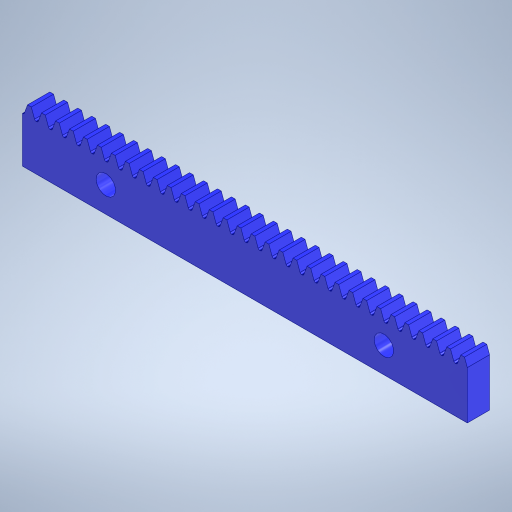
# Autodesk Inventor part: LRGEAM0.8KA-80-K2-B50
Saved by Autodesk Inventor 2024 (Build 280153000, 153)
## iProperties
Category: PARTsolutions
Company: MISUMI
Created: 2025-06-07
Part Number: LRGEAM0.8KA-80-K2-B50
Material: ナイロン 6
Catalog Web Link: www.cadenas.de
Description: LRGEA, LRGEAS,LRGEAB,LRGEAM,LRGEAP-Rack Gears L Dimension Configurable (One End Machined) - Pressure Angle 20 - Hole Qty. Configurable
Vendor: MISUMI
Document SubType Name: Modeling
Designer: psAdmin
Manufacturer: MISUMI
Mass: 3.19789 g
Surface Area: 25.3066 cm^2
Volume: 2.85525 cm^3
Density: 1.12 g/cm^3
Appearance: 青 - 壁塗料 - 光沢
PSOL_IDENT_0: {$CADENAS_DATA/23d-libs/misumi/metric/54_spur_gears/lrgea.prj},252 {VTYP=3D},{NB=LRGEAM0.8KA-80-K2-B
PSOL_IDENT_1: 50},{LINA=LRGEAM0.8KA-80-K2-B50},{NN=LRGEA, LRGEAS,LRGEAB,LRGEAM,LRGEAP},{DATE=29.05.2023 09:31:19},
PSOL_IDENT_2: {GEOMDATE=04.08.2020 02:33:51},{VERSION=},{LINEID=80},{WBVAR=MAT,L,HM,K,B,ALT1,ALT2,MS,ALT3,TPC},{WB
PSOL_IDENT_3: NUMERIC=L,K,B,MS}  {NB=LRGEAM0.8KA-80-K2-B50},{LINA=LRGEAM0.8KA-80-K2-B50},{KT=DUMMY},{PN=LRGEAM0.8K
PSOL_IDENT_4: A-80-K2-B50},{MAT=4},{MATALG='1','Free-Cutting Brass Bar','2','1045 Carbon Steel Equivalent','3','30
PSOL_IDENT_5: 4 Stainless Steel','4','MC Nylon','5','Polyacetal' },{TYPE=LRGEAM},{MOD=0.8},{MOD1=0.8},{L=80},{LALG=
PSOL_IDENT_6: [20:280/1]},{HM=KA},{HMALG='N','No Hole Machining','KA','Side Through Hole'},{K=2},{KALG=2},{DD21=1}
PSOL_IDENT_7: ,{M12=0},{B=50},{BALG=[50:50/1]},{BMIN=50},{BMAX=50},{F=15},{PITCH=2.513},{W=4},{H=10},{HH=9.2},{DD1=
PSOL_IDENT_8: 3.5},{DD2=0.0},{Z1=0.0},{M=-},{M1=0},{ALT1= },{ALT1ALG= ' ', 'Not applicable' },{ALT2= },{ALT2ALG= '
PSOL_IDENT_9: ', 'Not applicable' },{MS=0},{MSALG=0},{ALT3=},{ALT3ALG= '','Not applicable' },{TPC=N/A},{TPCA= 'N/
PSOL_IDENT_10: A' },{MCPN=},{WMCPN=},{ALT3PN=},{BPN=-B50},{NHPN=-K2},{MSPN=},{KK=1},{TED=1.800},{SP=1.2565},{PFP=0.
PSOL_IDENT_11: 304},{HAP=0.8},{HFP=1},{DEG1=20},{NN=32},{L1=0.919426},{NN1=32}
NB: LRGEAM0.8KA-80-K2-B50
NN: LRGEA, LRGEAS,LRGEAB,LRGEAM,LRGEAP
NT: Rack Gears L Dimension Configurable (One End Machined) - Pressure Angle 20 - Hole Qty. Configurable
NBSYN: $PN.
LINA: LRGEAM0.8KA-80-K2-B50
CATALOG: Misumi
PN: LRGEAM0.8KA-80-K2-B50
MAT: MC Nylon
MOD: 0.8
L: 80
HM: Side Through Hole
K: 2
B: 50
PITCH: 2.513
W: 4
H: 10
HH: 9.2
DD1: 3.5
DD2: 0
Z1: 0
M: -
ALT1: Not applicable
ALT2: Not applicable
MS: 0
ALT3: Not applicable
TPC: N/A
SUPPLIER: MISUMI
ARTICLENO: LRGEAM0.8KA-80-K2-B50
BOMINFO: LRGEAM0.8KA-80-K2-B50
CREATOR: CADENAS GmbH
Title: LRGEAM0.8KA-80-K2-B50
Author: Cadenas PARTsolutions
Comments: Rack Gears L Dimension Configurable (One End Machined) - Pressure Angle 20 - Hole Qty. Configurable
Autodesk Inventor part; units mm, degrees
ref_plane "YZ Plane" through (0, 0, 0) normal (1, 0, 0) x (0, 1, 0)
ref_plane "XZ Plane" through (0, 0, 0) normal (0, 1, 0) x (-1, 0, 0)
ref_plane "XY Plane" through (0, 0, 0) normal (0, 0, 1) x (1, 0, 0)
sketch "Sketch_1" plane through (0, 0, 0) normal (0, 0, 1) x (1, 0, 0)
  line L0 (0, 10) -> (0, 0)
  line L1 (0, 0) -> (80, 0)
  line L2 (80, 0) -> (80, 10)
  line L3 (80, 10) -> (0, 10)
  constraints: 8 end point
extrude "Extrusion1" add sketch "Sketch_1" along normal blind 4
sketch "Sketch_21" plane through (0, 0, 0) normal (0, 0, 1) x (1, 0, 0)
  line L0 (-0.9194, 10) -> (-0.3371, 8.4)
  arc A0 (-0.3371, 8.4) -> (-0.0514, 8.2) centre (-0.0514, 8.504) ccw
  line L1 (-0.0514, 8.2) -> (0.0514, 8.2)
  arc A1 (0.0514, 8.2) -> (0.3371, 8.4) centre (0.0514, 8.504) ccw
  line L2 (0.3371, 8.4) -> (0.9194, 10)
  line L3 (0.9194, 10) -> (-0.9194, 10)
  constraints: 8 end point, 4 point on circle, 2 centre point
extrude "Extrusion2" cut sketch "Sketch_21" along normal blind 4
pattern_linear "Rectangular Pattern1" count 33 spacing 2.513 along (1, 0, 0) of "Extrusion2"
sketch "Sketch3" plane through (0, 0, 0) normal (0, 0, -1) x (-1, 0, 0)
  point P0 (-15, 4.6)
hole "Hole1" at (15, 4.6, 0) direction (0, 0, 1) diameter 3.5 depth 4
pattern_linear "Rectangular Pattern2" count 2 spacing 50 along (1, 0, 0) of "Hole1"
body "Solid1"
